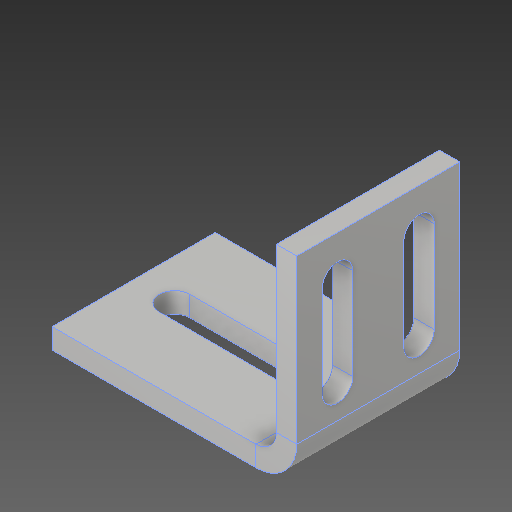
# Autodesk Inventor part: keyL_medium
Saved by Autodesk Inventor 2018 (Build 220112000, 112)
## iProperties
Created: 2018-05-26
Part Number: keyL_medium
Material: アルミニウム 6061
Document SubType Name: Sheet Metal
Designer: NaMACHAN
Density: 2.7 g/cm^3
Sheet Metal Rule: AL2mm
Appearance: アルミニウム - フラット
Mass: 2.91704 g
Surface Area: 14.8378 cm^2
Volume: 1.08038 cm^3
Author: NaMACHAN
Autodesk Inventor part; units mm, degrees
ref_plane "YZ Plane" through (0, 0, 0) normal (1, 0, 0) x (0, 1, 0)
ref_plane "XZ Plane" through (0, 0, 0) normal (0, 1, 0) x (-1, 0, 0)
ref_plane "XY Plane" through (0, 0, 0) normal (0, 0, 1) x (1, 0, 0)
sketch "スケッチ1" plane through (0, 0, 0) normal (0, 1, 0) x (-1, 0, 0)
  line L0 (-10, 8) -> (10, 8)
  line L1 (10, 8) -> (10, -8)
  line L2 (10, -8) -> (-10, -8)
  line L3 (-10, -8) -> (-10, 8)
  line L4 (-10, 8) -> (10, -8) construction
  line L5 (10, 8) -> (-10, -8) construction
  point P0 (0, 0)
  dimension "d0" = 20
  dimension "d1" = 16
  measures "d0" distance of L1.end L2.end
  measures "d1" distance of L0.end L1.end
extrude "プレート1" add sketch "スケッチ1" along normal blind 2
sketch "スケッチ2" plane through (12, 4, -8) normal (1, 0, 0) x (0, 1, 0)
  line L0 (0, 16) -> (0, 0)
  line L1 (0, 0) -> (16, 0)
  line L2 (16, 0) -> (16, 16)
  line L3 (16, 16) -> (0, 16)
  constraints: 6 end point, 1 horizontal, 1 perpendicular, 1 vertical
edge flange "フランジ1" height 20 angle 90 thickness 2 bend radius 2 thickness toward (1, 0, 0) relief tear relief width 2 relief depth 1 edges at (10, 2, 0) wall of the first edge with corners at (12, 4, 8) (12, 4, -8) (12, 20, -8) (12, 20, 8)
bend "曲げ1"
corner "コーナー1"
sketch "スケッチ3" plane through (14, 20, 8) normal (1, 0, 0) x (0, 0, -1)
  line L0 (2.5, -4) -> (2.5, -13)
  arc A0 (2.5, -13) -> (5.5, -13) centre (4, -13) ccw
  line L1 (5.5, -13) -> (5.5, -4)
  arc A1 (5.5, -4) -> (2.5, -4) centre (4, -4) ccw
  line L2 (10.5, -4) -> (10.5, -13)
  arc A2 (10.5, -13) -> (13.5, -13) centre (12, -13) ccw
  line L3 (13.5, -13) -> (13.5, -4)
  arc A3 (13.5, -4) -> (10.5, -4) centre (12, -4) ccw
  line L4 (0, -16) -> (0, 0) projected
  line L5 (16, 0) -> (16, -16) projected
  line L6 (0, 0) -> (16, 0) projected
  line L7 (0, -16) -> (16, -16) projected
  point P0 (8, -20)
  dimension "d13" = 4
  dimension "d14" = 4
  dimension "d17" = 3
  dimension "d18" = 4
  dimension "d19" = 1.5
  dimension "d20" = 1.5
  constraints: 8 end point, 8 point on circle, 8 tangent, 4 centre point, 2 horizontal alignment, 2 parallel, 2 vertical
  measures "d13" distance from line of L4 A1.centre
  measures "d14" distance from line of L5 A3.centre
  measures "d17" distance from line of L7 A2.centre
  measures "d18" distance from line of A3.centre L6
  measures "d19" radius of A3
  measures "d20" radius of A1
extrude "押し出し1" cut sketch "スケッチ3" against normal blind 10 contours A1 L1 A0 L0 | A3 L3 A2 L2
sketch "スケッチ4" plane through (0, 2, 0) normal (0, 1, 0) x (1, 0, 0)
  line L0 (-6, -1.5) -> (6, -1.5)
  arc A0 (6, -1.5) -> (6, 1.5) centre (6, 0) ccw
  line L1 (6, 1.5) -> (-6, 1.5)
  arc A1 (-6, 1.5) -> (-6, -1.5) centre (-6, 0) ccw
  line L2 (-10, -8) -> (-10, 8) projected
  line L3 (10, 8) -> (10, -8) projected
  point P0 (0, 0)
  dimension "d23" = 4
  dimension "d24" = 4
  dimension "d25" = 1.5
  constraints: 4 end point, 4 point on circle, 4 tangent, 2 centre point, 1 horizontal, 1 horizontal alignment, 1 parallel
  measures "d23" distance from line of L2 A1.centre
  measures "d24" distance from line of L3 A0.centre
  measures "d25" radius of A1
extrude "押し出し2" cut sketch "スケッチ4" against normal blind 10
equation "\"d2\" = Thickness"
equation "\"d3\" = BendReliefWidth"
equation "\"d4\" = BendReliefDepth"
equation "\"d5\" = MinimumRemnant"
equation "\"d6\" = TransitionRadius"
equation "\"d9\" = BendRadius"
equation "\"d10\" = CornerReliefSize"
equation "\"d11\" = GapSize"
equation "\"d12\" = JacobiRadiusSize"
equation "\"BendRadius\" = Thickness"
equation "\"BendReliefWidth\" = Thickness"
equation "\"BendReliefDepth\" = 0.5 * Thickness"
equation "\"CornerReliefSize\" = 4 * Thickness"
equation "\"MinimumRemnant\" = 2 * Thickness"
equation "\"TransitionRadius\" = BendRadius"
equation "\"JacobiRadiusSize\" = BendRadius"
equation "\"GapSize\" = Thickness"
equation "\"Thickness\" = 2"
